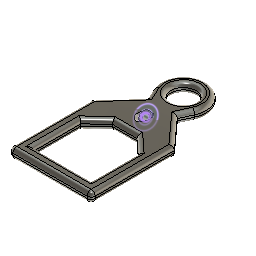
RT24_CapsLock (Autodesk Fusion 360 design; units mm, degrees)
Autodesk Fusion 360 part; units mm, degrees
sketch "Sketch1" plane through (0, 0, 0) normal (0, 0, 1) x (1, 0, 0)
  line L0 (11.5, 12.5) -> (-11.5, 12.5)
  line L1 (-11.5, 12.5) -> (-11.5, -12.5)
  line L2 (-11.5, -12.5) -> (11.5, -12.5)
  line L3 (11.5, -12.5) -> (11.5, 12.5)
  line L4 (11.5, 12.5) -> (-11.5, -12.5) construction
  line L5 (-11.5, 12.5) -> (11.5, -12.5) construction
  line L6 (0, 38) -> (0, -20) construction
  line L7 (0, 27.5) -> (-6, 27.5)
  line L8 (16.5, -17.5) -> (16.5, 17.5)
  line L9 (16.5, 17.5) -> (-16.5, 17.5)
  line L10 (-16.5, 17.5) -> (-16.5, -17.5)
  line L11 (-16.5, -17.5) -> (16.5, -17.5)
  line L12 (-6, 27.5) -> (-16.5, 15.8333)
  line L13 (0, 27.5) -> (6, 27.5)
  line L14 (6, 27.5) -> (16.5, 15.8333)
  line L15 (-4.8766, 12.5) -> (-11.5, 6.4065)
  line L16 (4.8766, 12.5) -> (11.5, 6.4065)
  circle A0 centre (0, 36) radius 5
  circle A1 centre (0, 36) radius 9
  line L17 (0, 24.036) -> (-17, 24.036) construction
  line L18 (-6, 27.5) -> (-8.1787, 32.2438)
  line L19 (6, 27.5) -> (8.1787, 32.2438)
  point P0 (0, 24.036)
  dimension "d1" = 23
  dimension "d2" = 25
  dimension "d7" = 40
  dimension "d8" = 5
  dimension "d9" = 36.536
  dimension "d10" = 9
  dimension "d11" = 10
  dimension "d12" = 4
  constraint horizontal L0
  constraint perpendicular L0 L1
  constraint parallel L0 L2
  constraint parallel L1 L3
  constraint coincident L4 origin
  constraint coincident L5 origin
  constraint perpendicular L2 L6
  constraint coincident L6 L7.start
  constraint perpendicular L6 L7
  constraint coincident L10 L12.end
  constraint symmetric L6 L7.start L13.start
  constraint symmetric L6 L7.end L13.end
  constraint symmetric L6 L12.end L14.end
  constraint coincident L0 L15.start
  constraint coincident L1 L15.end
  constraint perpendicular L5 L15
  constraint symmetric L6 L15.start L16.start
  constraint symmetric L6 L15.end L16.end
  constraint coincident P0 L17.start
  constraint perpendicular L6 L17
  constraint coincident L6 A0.centre
  constraint coincident A1 L18.end
  constraint tangent A1 L18
  constraint coincident A1 L19.end
  constraint tangent A1 L19
  measures "d1" distance of L1.end L2.end
  measures "d2" distance of L0.end L1.end
  measures "d7" distance of L2 L7
  measures "d9" distance of L2 P0
  measures "d10" distance of L15.start L15.end
  measures "d11" diameter of A0
extrude "Extrude1" add sketch "Sketch1" along normal blind 4 contours L0 L3 L16 | L0 L1 L15 | L7 L13 A1 | L7 L13 A1 | L7 L9 L12 L13 L14 A1 | L7 A1 L18 | L13 A1 L19 | L8 L9 L10 L11 L12 L14
ref_plane "WorkPlane1" through (-8.5, 24.036, 0) normal (0, -0.707107, 0.707107) x (-1, 0, 0)
sketch "Sketch2" plane through (-8.5, 24.036, 0) normal (0, -0.707107, 0.707107) x (-1, 0, 0)
  circle A0 centre (-8.5, 0) radius 1.2
  circle A1 centre (-8.5, 0) radius 2.25
  circle A2 centre (-8.5, 0) radius 4
  point P0 (-8.5, 0)
  dimension "d16" = 2.4
  dimension "d17" = 4.5
  dimension "d18" = 8
  constraint coincident P0 A0.centre
  constraint concentric A0 A1
  measures "d16" diameter of A0
  measures "d17" diameter of A1
  measures "d18" diameter of A2
extrude "Extrude2" cut sketch "Sketch2" along normal through all and the other way blind 7.753 contours A0
ref_plane "WorkPlane2" through (0, 20.854, 3.182) normal (0, -0.707107, 0.707107) x (-1, 0, 0)
sketch "Sketch3" plane through (0, 20.854, 3.182) normal (0, -0.707107, 0.707107) x (-1, 0, 0)
  circle A0 centre (0, 0) radius 1.2
  circle A1 centre (0, 0) radius 2.25
  circle A2 centre (0, 0) radius 4
extrude "Extrude4" cut sketch "Sketch3" along normal blind 10.1125 contours A1
extrude "Extrude6" add sketch "Sketch3" against normal blind 1.187 contours A1
fillet "Fillet1" radius 1.6 31 edges at (0, 45, 4) (-7.0893, 29.8719, 4) (7.0893, 29.8719, 4) (-4.6616, 37.8081, 4) (-4.6616, 37.8081, 0) (0, 45, 0) (-7.0893, 29.8719, 0) (7.0893, 29.8719, 0) (-11.25, 21.6667, 4) (-16.5, -0.8333, 4) (-16.5, -0.8333, 0) (0, -17.5, 4) (0, -17.5, 0) (16.5, -0.8333, 4) (16.5, -0.8333, 0) (-8.1883, 9.4532, 4) (0, 12.5, 4) (-11.5, -3.0468, 4) (0, -12.5, 4) (11.5, -3.0468, 4) (8.1883, 9.4532, 4) (11.5, -3.0468, 0) (0, -12.5, 0) (-11.5, -3.0468, 0) (0, 12.5, 0) (-8.1883, 9.4532, 0) (8.1883, 9.4532, 0) (11.25, 21.6667, 4) (11.25, 21.6667, 0) (16.5, -17.5, 2) (-16.5, -17.5, 2)
